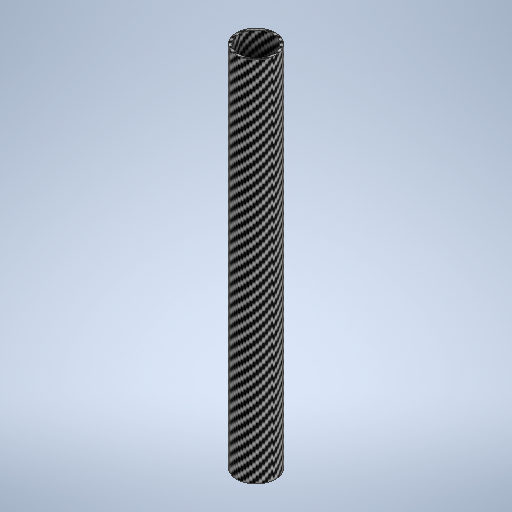
# Autodesk Inventor part: Carbon Fiber Round Tube 330x16x14mm
Saved by Autodesk Inventor 2026.2 (Build 302298010, 298A)
## iProperties
Created: 2026-03-12
Part Number: Carbon Fiber Round Tube 330x16x14mm
Material: PET Plastic
Document SubType Name: Modeling
Designer: tngzj
Density: 1.541 g/cm^3
Appearance: Carbon Fiber
Mass: 23.9639 g
Surface Area: 311.96 cm^2
Volume: 15.5509 cm^3
Author: tngzj
Autodesk Inventor part; units mm, degrees
ref_plane "YZ Plane" through (0, 0, 0) normal (1, 0, 0) x (0, 1, 0)
ref_plane "XZ Plane" through (0, 0, 0) normal (0, 1, 0) x (-1, 0, 0)
ref_plane "XY Plane" through (0, 0, 0) normal (0, 0, 1) x (1, 0, 0)
sketch "Sketch1" plane through (0, 0, 0) normal (0, 1, 0) x (-1, 0, 0)
  circle A0 centre (0, 0) radius 7
  circle A1 centre (0, 0) radius 8
  dimension "d0" = 14
  dimension "d1" = 16
  constraints: 2 centre point, 2 coincident
  measures "d0" diameter of A0
  measures "d1" diameter of A1
extrude "Extrusion1" add sketch "Sketch1" along normal blind 150
body "Solid1"
